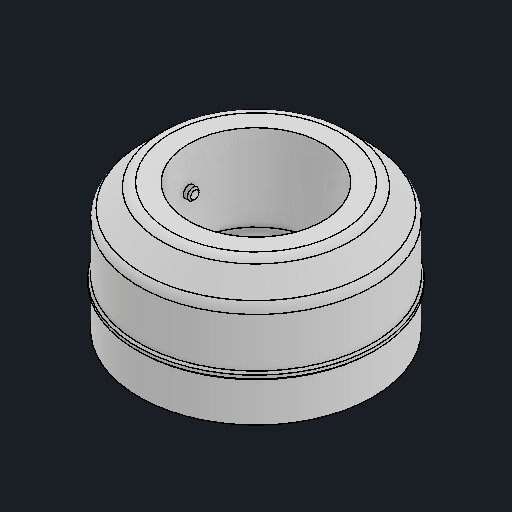
# Autodesk Inventor part: Cyclone Hose Adapter
Saved by Autodesk Inventor 2026.2 (Build 302298000, 298)
## iProperties
Created: 2026-06-17
Part Number: Cyclone Hose Adapter
Material: Generic
Document SubType Name: Modeling
Designer: JoshuaEah
Density: 1 g/cm^3
Appearance: Default
Author: JoshuaEah
Autodesk Inventor part; units mm, degrees
ref_plane "YZ Plane" through (0, 0, 0) normal (1, 0, 0) x (0, 1, 0)
ref_plane "XZ Plane" through (0, 0, 0) normal (0, 1, 0) x (-1, 0, 0)
ref_plane "XY Plane" through (0, 0, 0) normal (0, 0, 1) x (1, 0, 0)
sketch "Sketch1" plane through (0, 0, 0) normal (0, 1, 0) x (-1, 0, 0)
  circle A0 centre (0, 0) radius 16.2
  circle A1 centre (0, 0) radius 28.25
  circle A2 centre (0, 0) radius 28.75
  line L0 (17.6, 1.4) -> (14.8, 1.4)
  line L1 (14.8, 1.4) -> (14.8, -1.4)
  line L2 (14.8, -1.4) -> (17.6, -1.4)
  line L3 (17.6, -1.4) -> (17.6, 1.4)
  line L4 (17.6, 1.4) -> (14.8, -1.4) construction
  line L5 (14.8, 1.4) -> (17.6, -1.4) construction
  line L6 (16.2, 0) -> (14.8, 0)
  line L7 (16.2, 1.4) -> (16.2, -1.4)
  circle A3 centre (0, 0) radius 11
  point P0 (16.1394, -1.4)
  point P1 (16.2, 0)
  dimension "d0" = 32.4
  dimension "d1" = 56.5
  dimension "d12" = 0.5
  dimension "d20" = 2.8
  dimension "d21" = 2.8
  dimension "d26" = 22
  constraints: 16 end point, 5 midpoint, 4 coincident, 3 centre point, 2 parallel, 1 horizontal, 1 horizontal alignment, 1 perpendicular, 3 other
  measures "d1" diameter of A1
  measures "d12" radial gap between concentric circles of A2 A1
  measures "d20" distance of L2.end L1.end
  measures "d21" distance of L1.end L0.end
  measures "d26" diameter of A3
extrude "Top" add sketch "Sketch1" along normal blind 10 contours L7 L2 A0 | A0 L0 L7 | L7 L0 L3 L2 | A1
extrude "Middle" add sketch "Sketch1" against normal blind 10 contours L7 L2 A0 | A0 L0 L7 | L7 L0 L3 L2 | A1
extrude "Outer Ring" add sketch "Sketch1" against normal blind 0.8 from surface at -10 contours L7 L2 A0 | A0 L0 L7 | L7 L0 L3 L2 | A1 | A2
extrude "Bottom" add sketch "Sketch1" against normal blind 10 from surface at -10.8 contours L6 L1 L0 A0 | L7 L2 A0 | A0 L2 L1 L6 | A0 L0 L7 | L7 L0 L3 L2 | L0 L1 L2 A0 | A1
revolve "Cam" add sketch "Sketch1" angle 360 about axis through (-16.2, 0, 0) along (1, 0, 0) contours L7 L2 A0 | A0 L2 L1 L6
chamfer "Cam Chamfer" distance 0.4 angle 45 1 edges at (-14.8, 0, 1.4)
chamfer "Chamfer1" distance 6.35 angle 45 1 edges at (28.25, 10, 0)
fillet "Fillet1" radius 3.175 2 edges at (21.9, 10, 0) (28.25, 3.65, 0)
chamfer "Chamfer2" distance 0.5 angle 45 2 edges at (28.25, -10.8, 0) (28.25, -10, 0)
body "Solid1"
